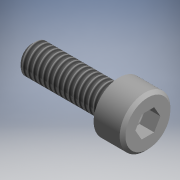
# Autodesk Inventor part: M4-12_bo2
Saved by Autodesk Inventor 2017.3 (Build 213256000, 256)
## iProperties
Part Number: M4-12_bo2
Material: Generic
Catalog Web Link: www.cadenas.de
Description: Screw_b2-Couplings - Hexagon Socket Head Cap Screw
Vendor: MISUMI
Document SubType Name: Modeling
Designer: partserver
Manufacturer: MISUMI
Mass: 0.284447 g
Surface Area: 3.27785 cm^2
Volume: 0.284447 cm^3
Density: 1 g/cm^3
Appearance: PSOLRGB-192-192-192
Category: PARTsolutions
Company: MISUMI
Title: M4-12
Author: Cadenas PARTsolutions
Comments: Couplings - Hexagon Socket Head Cap Screw
PSOL_IDENT_0: {$CADENAS_DATA\23d-libs\misumi\metric\50_couplings\parts\screw_mcocwk.prj},159 {VTYP=3D},{NB=M4-12_b
PSOL_IDENT_1: o2},{LINA=M4-12},{NN=Screw_b2},{DATE=30.03.2018 07:24:47},{GEOMDATE=14.04.2017 04:57:00},{VERSION=},
PSOL_IDENT_2: {LINEID=290},{WBVAR=L},{WBNUMERIC=L}  {NB=M4-12_bo2},{LINA=M4-12},{KT=DUMMY},{PN=M4-12},{M=M4},{THMD
PSOL_IDENT_3: 1=4.0000},{THMIN1=3.2420},{KK=4.00},{L=12},{LALG=12,16},{DK=7.0},{S=3.00},{TT=2.0},{EE=3.44},{DA=4.7
PSOL_IDENT_4: },{DS=4.0},{VV=0.40},{RR=0.2},{IT=0.65645}
NB: M4-12_bo2
NN: Screw_b2
NT: Couplings - Hexagon Socket Head Cap Screw
NBSYN: $PN._bo2
LINA: M4-12
CATALOG: Misumi
PN: M4-12
M: M4
KK: 4
L: 12
DK: 7
S: 3
TT: 2
EE: 3.44
DA: 4.7
DS: 4
VV: 0.4
RR: 0.2
SUPPLIER: MISUMI
ARTICLENO: M4-12_bo2
BOMINFO: M4-12
CREATOR: CADENAS GmbH
Autodesk Inventor part; units mm, degrees
sketch "Sketch_1" plane through (0, 0, 0) normal (0, 0, 1) x (1, 0, 0)
  line L0 (12, 0) -> (-4, 0)
  line L1 (-4, 0) -> (-4, 3.1)
  line L2 (-4, 3.1) -> (-3.6, 3.5)
  line L3 (-3.6, 3.5) -> (0, 3.5)
  line L4 (0, 3.5) -> (0, 2.2)
  arc A0 (0, 2.2) -> (0.2, 2) centre (0.2, 2.2) ccw
  line L5 (0.2, 2) -> (11.5705, 2)
  line L6 (11.5705, 2) -> (12, 1.5705)
  line L7 (12, 1.5705) -> (12, 0)
  line L8 (12, 0) -> (-4, 0)
  constraints: 18 end point, 2 point on circle, 1 centre point
revolve "Revolution1" add sketch "Sketch_1" angle 360 about axis through (12, 0, 0) along (1, 0, 0)
thread "Thread1" size "M4x0.7" class "6g" standard "ISO Metric profile" length 10.714
sketch "Sketch_2" plane through (-4, 0, 0) normal (1, 0, 0) x (0, 0, -1)
  line L0 (-1.5, -0.866) -> (0, -1.7321)
  line L1 (0, -1.7321) -> (1.5, -0.866)
  line L2 (1.5, -0.866) -> (1.5, 0.866)
  line L3 (1.5, 0.866) -> (0, 1.7321)
  line L4 (0, 1.7321) -> (-1.5, 0.866)
  line L5 (-1.5, 0.866) -> (-1.5, -0.866)
  constraints: 12 end point
extrude "Extrusion1" cut sketch "Sketch_2" along normal blind 2
sketch "Sketch_5" plane through (0, 0, 0) normal (0, 0, 1) x (1, 0, 0)
  line L0 (-1.134, 0) -> (-2, 0)
  line L1 (-2, 0) -> (-2, 1.5)
  line L2 (-2, 1.5) -> (-1.134, 0)
  line L3 (-1.134, 0) -> (-2, 0)
  constraints: 8 end point
revolve "Revolution2" cut sketch "Sketch_5" angle 360 about axis through (-1.134, 0, 0) along (1, 0, 0)
ref_plane "SCW_XY" through (0, 0, 0) normal (1, 0, 0) x (0, 0, -1)
ref_plane "SCW_YZ" through (0, 0, 0) normal (0, 0, -1) x (0, 1, 0)
ref_plane "SCW_ZX" through (0, 0, 0) normal (0, 1, 0) x (1, 0, 0)
body "Solid1"
